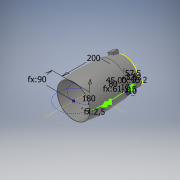
# Autodesk Inventor part: Form
Saved by Autodesk Inventor 2019.1 (Build 231200000, 200)
## iProperties
Created: 2018-07-22
Part Number: Form
Material: Generisch
Document SubType Name: Modeling
Designer: JochenAlt
Density: 1 g/cm^3
Appearance: Textur - grau
Author: JochenAlt
Autodesk Inventor part; units mm, degrees
ref_plane "YZ Plane" through (0, 0, 0) normal (1, 0, 0) x (0, 1, 0)
ref_plane "XZ Plane" through (0, 0, 0) normal (0, 1, 0) x (-1, 0, 0)
sketch "Skizze3" plane through (0, 0, 0) normal (0, 0, 1) x (1, 0, 0)
  line L0 (0, 280.2532) -> (0, -256.7089) construction
  line L1 (-139.25, 0) -> (205.5, 0) construction
  circle A0 centre (0, 0) radius 90 construction
  circle A1 centre (0, -90) radius 90 construction
  line L2 (93, -90) -> (95.5, -90)
  line L3 (97.3301, 125.8581) -> (106.556, 4.4565) construction
  line L4 (106.556, -20.4324) -> (95.5, -90) construction
  spline S0 degree 3 poles (97.3301, 125.8581) (106.556, 4.4565) (106.556, -20.4324) (95.5, -90) knots 1 1 1 1 2 2 2 2
  line L5 (153.75, 101.6438) -> (156.25, 101.6438) construction
  line L6 (106.556, 4.4565) -> (106.556, -20.4324) construction
  line L7 (63.6396, 63.6396) -> (107.1267, 107.1267) construction
  line L8 (63.6396, -26.3604) -> (107.1267, 17.1267) construction
  circle A2 centre (107.1267, 17.1267) radius 8.5 construction
  circle A3 centre (107.1267, 107.1267) radius 8.5 construction
  line L9 (93, -90) -> (90, -90) construction
  line L10 (115.2082, 109.7607) -> (119.9621, 111.3102) construction
  arc A4 (109.3117, 123.4538) -> (109.3117, 144.667) centre (98.7051, 134.0604) ccw construction
  line L11 (109.3117, 123.4538) -> (65.9557, 80.0979) construction
  line L12 (97.3301, 125.8581) -> (95.9974, 143.3954) construction
  line L13 (95.9974, 143.3954) -> (82.5, 200) construction
  spline S1 degree 2 poles (97.3301, 125.8581) (95.9974, 143.3954) (82.5, 200) knots 1 1 1 2 2 2
  line L14 (82.5, 200) -> (80, 200)
  line L15 (106.556, 4.4565) -> (104.056, 4.4565) construction
  line L16 (93, -90) -> (104.056, -20.4324) construction
  line L17 (104.056, -20.4324) -> (104.056, 4.4565) construction
  line L18 (104.056, 4.4565) -> (99.287, 134.9562) construction
  line L19 (99.287, 134.9562) -> (80, 200) construction
  spline S2 degree 4 poles (93, -90) (104.056, -20.4324) (104.056, 4.4565) (99.287, 134.9562) (80, 200) knots 1 1 1 1 1 2 2 2 2 2
  line L20 (106.556, -20.4324) -> (104.056, -20.4324) construction
  line L21 (103.1815, 36.8961) -> (100.6832, 36.8033) construction
  line L22 (100.4819, 82.7242) -> (97.9898, 82.5262) construction
  line L23 (80, 200) -> (-80, 200) construction
  line L24 (-80, 113.6868) -> (80, 113.6868) construction
  dimension "d13" = 180
  dimension "d108" = 17
  dimension "d14" = 90
  dimension "d18" = 2.5
  dimension "d106" = 61.5
  dimension "d107" = 45
  dimension "d110" = 3
  dimension "d112" = 5
  dimension "d119" = 10
  dimension "d120" = 15
  dimension "d203" = 80
  dimension "d204" = 200
  constraints: 28 end point, 7 equal length, 7 horizontal, 6 coincident, 5 point on circle, 3 centre point, 3 point on line, 2 parallel, 2 symmetric about line, 1 collinear, 1 line through centre, 1 tangent, 1 vertical, 24 other
  measures "d14" distance of A1.centre point (0, 0)
  measures "d18" distance of L2.end L2.start
  measures "d106" distance of L7.start L7.end
  measures "d107" angle of L0 L7
  measures "d110" distance of L2.start L9.end
  measures "d112" distance of L10.start L10.end
  measures "d119" distance from line of L11.start L7
  measures "d120" radius of A4
  measures "d203" distance from line of L0 L14.end
  measures "d204" distance from line of L23 point (0, 0)
revolve "Umdrehung1" add sketch "Skizze3" angle 360 about axis through (0, 0, 0) along (0, -1, 0)
ref_plane "Arbeitsebene3" through (80, 200, 0) normal (0, 1, 0) x (-1, 0, 0)
sketch "Skizze7" plane through (0, 200, 0) normal (0, 1, 0) x (-1, 0, 0)
  line L0 (-55.8972, -9.4653) -> (-75.4587, -12.7777)
  line L1 (-55.8972, 9.4653) -> (-90.142, 15.264)
  line L2 (-97.3301, 0) -> (-104.0363, 0) construction
  arc A0 (-55.8972, -9.4653) -> (-55.8972, 9.4653) centre (-57.5, 0) ccw
  circle A1 centre (-57.5, 0) radius 5.1
  line L3 (-75.4587, -12.7777) -> (-99.8278, -16.9042)
  line L4 (-90.142, 15.264) -> (-99.8278, 16.9042)
  line L5 (0, -115.5) -> (0, 115.5) construction
  line L6 (-37.4, -64.7787) -> (-37.4, -64.7787)
  arc A2 (-70.3446, -10.6589) -> (-70.3446, -10.6589) centre (0, 0) ccw
  arc A3 (-59, -7.4505) -> (-56, -7.4505) centre (-57.5, 0) ccw
  arc A4 (-56, 7.4505) -> (-59, 7.4505) centre (-57.5, 0) ccw
  arc A5 (-56, -5.9127) -> (-56, 5.9127) centre (-57.5, 0) ccw
  arc A6 (-59, 5.9127) -> (-59, -5.9127) centre (-57.5, 0) ccw
  line L7 (-56, -7.4505) -> (-56, -5.9127)
  line L8 (-56, 5.9127) -> (-56, 7.4505)
  line L9 (-59, -7.4505) -> (-59, -5.9127)
  line L10 (-59, 5.9127) -> (-59, 7.4505)
  line L11 (-57.5, -7.6) -> (-57.5, 7.6) construction
  arc A7 (-99.8278, 16.9042) -> (-99.8278, -16.9042) centre (0, 0) ccw construction
  arc A8 (-100.1327, 16.9558) -> (-100.1327, -16.9558) centre (0, 0) ccw
  line L12 (-100.1327, -16.9558) -> (-99.8278, -16.9042)
  line L13 (-100.1327, 16.9558) -> (-99.8278, 16.9042)
  circle A9 centre (0, 0) radius 80 projected
  circle A10 centre (0, 0) radius 82.5 projected
  point P0 (-95.5, 0)
  point P1 (-104.0582, 0)
  point P2 (-101.2489, 0)
  dimension "d142" = 57.5
  dimension "d196" = 12.2
  dimension "d197" = 1
  dimension "d199" = 3
  dimension "d200" = 15.2
  dimension "d201" = 3.5
  constraints: 24 end point, 20 point on circle, 9 centre point, 6 collinear, 5 vertical, 4 coincident, 3 concentric, 3 point on line, 2 tangent, 1 equal length, 1 midpoint, 2 other
  measures "d142" distance of A0.centre point (0, 0)
  measures "d196" diameter of A5
  measures "d197" radial gap between concentric circles of A1 A5
  measures "d199" distance between parallel lines of L9 L7
  measures "d200" diameter of A3
  measures "d201" radial gap between concentric circles of A0 A5
extrude "Extrusion5" add sketch "Skizze7" against normal blind 30 separate body contours L0 A2 L1 A0 | L0 L3 A9 L1 A2 | L3 A10 L1 A9 | L3 L12 A8 L13 L4 L1 A10 picked at (-67.9054, -6.4348) picked at (-76.9288, -1.3254) picked at (-80.8634, -10.5803)
extrude "Extrusion8" add sketch "Skizze7" along normal blind 2 from surface at 0 contours L9 A6 L10 A4 L8 A5 L7 A3 bodies 2
pattern_circular "Runde Anordnung2" count 3 over 360 about axis through (0, -10, 0) along (0, 1, 0) bodies 2
equation "\"d14\" = 0.5 * d13"
equation "\"d18\" = d17"
equation "\"d16\" = d11"
equation "\"d17\" = d16"
equation "\"d11\" = 2.5"
